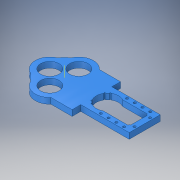
# Autodesk Inventor part: 000.401 - Опорная платформа
Saved by Autodesk Inventor 2019 (Build 230136000, 136)
## iProperties
Created: 2020-03-18
Part Number: 000.401 - Опорная платформа
Material: Пластик АБС
Document SubType Name: Modeling
Designer: Петров Иван
Density: 1.06 g/cm^3
Appearance: Голубой
Author: Петров Иван
Autodesk Inventor part; units mm, degrees
ref_plane "YZ Plane" through (0, 0, 0) normal (1, 0, 0) x (0, 1, 0)
ref_plane "XZ Plane" through (0, 0, 0) normal (0, 1, 0) x (-1, 0, 0)
ref_plane "XY Plane" through (0, 0, 0) normal (0, 0, 1) x (1, 0, 0)
sketch "Эскиз1" plane through (0, 0, 0) normal (0, 1, 0) x (-1, 0, 0)
  circle A0 centre (0, 0) radius 13.8
  circle A1 centre (-8, 0) radius 1.2
  circle A2 centre (0, -8) radius 1.2
  circle A3 centre (8, 0) radius 1.2
  circle A4 centre (0, 8) radius 1.2
  circle A5 centre (-7.7782, 7.7782) radius 1.2813
  circle A6 centre (-11, 0) radius 1.2813
  circle A7 centre (-7.7782, -7.7782) radius 1.2813
  circle A8 centre (0, -11) radius 1.2812
  circle A9 centre (7.7782, -7.7782) radius 1.2812
  circle A10 centre (11, 0) radius 1.2813
  circle A11 centre (7.7782, 7.7782) radius 1.2812
  circle A12 centre (0, 11) radius 1.2812
  circle A13 centre (0, 0) radius 5
  circle A14 centre (0, 0) radius 14
  circle A15 centre (0, 0) radius 1.55
  circle A16 centre (0, 0) radius 1.75
  circle A17 centre (0, 0) radius 25
  dimension "d0" = 50
  constraints: 18 centre point, 1 coincident
  measures "d0" diameter of A17
extrude "Выдавливание1" add sketch "Эскиз1" along normal blind 6 contours A0 | A1 | A2 | A3 | A4 | A5 | A6 | A7 | A8 | A9 | A10 | A11 | A12 | A13 | A14 | A15 | A16 | A17
sketch "Эскиз2" plane through (0, 6, 0) normal (0, 1, 0) x (1, 0, 0)
  line L0 (25, 0) -> (100, 0)
  circle A0 centre (100, 0) radius 25
  line L1 (50, 0) -> (50, -20)
  line L2 (50, 0) -> (50, 20)
  circle A1 centre (0, 0) radius 25 projected
  arc A2 (4.9455, 24.506) -> (95.0545, 24.506) centre (50, 247.5) ccw
  arc A3 (95.0545, -24.506) -> (4.9455, -24.506) centre (50, -247.5) ccw
  line L3 (100, 25) -> (0, 25)
  line L4 (0, -25) -> (100, -25)
  line L5 (50, 20) -> (50, 25)
  line L6 (50, -20) -> (50, -25)
  line L7 (50, 25) -> (50, -25)
  dimension "d3" = 100
  dimension "d4" = 50
  dimension "d5" = 20
  dimension "d6" = 20
  constraints: 16 end point, 15 point on circle, 3 centre point, 3 tangent, 2 midpoint, 2 vertical, 1 coincident, 1 collinear, 1 horizontal, 1 point on line
  measures "d3" distance of point (0, 0) L0.end
  measures "d4" diameter of A0
  measures "d5" distance of L1.start L1.end
  measures "d6" distance of L1.start L2.end
extrude "Выдавливание2" add sketch "Эскиз2" against normal blind 6 contours A1 A2 L2 L0 | L0 L1 A3 A1 | A1 L3 L5 A2 | A3 L6 L4 A1
sketch "Эскиз7" plane through (0, 6, 0) normal (0, 1, 0) x (1, 0, 0)
  line L0 (100, 0) -> (100, 15)
  line L1 (100, 0) -> (100, -15)
  circle A0 centre (100, 15) radius 3
  circle A1 centre (100, -15) radius 3
  line L2 (100, 0) -> (115, 0)
  circle A2 centre (115, 0) radius 3
  point P0 (0, 0)
  dimension "d23" = 15
  dimension "d24" = 15
  dimension "d25" = 6
  dimension "d26" = 6
  dimension "d27" = 15
  dimension "d28" = 6
  constraints: 6 end point, 3 centre point, 3 coincident, 2 vertical, 1 horizontal, 1 other
  measures "d23" distance of L0.start L0.end
  measures "d24" distance of L0.start L1.end
  measures "d25" diameter of A0
  measures "d26" diameter of A1
  measures "d27" distance of L0.start L2.end
  measures "d28" diameter of A2
extrude "Выдавливание7" [suppressed]
move faces "Перенос1" translate (33, 0, 0) faces at (50, 4, 8.3333)
sketch "Эскиз11" plane through (0, 6, 0) normal (0, 1, 0) x (1, 0, 0)
  line L0 (83, -25) -> (0, -25) projected
  line L1 (83, -25) -> (33, -25)
  line L2 (33, -25) -> (33, -16)
  line L3 (33, -16) -> (83, -16)
  line L4 (83, -16) -> (83, -25)
  point P0 (0, 0)
  dimension "d41" = 50
  dimension "d42" = 9
  constraints: 8 end point, 2 parallel, 1 horizontal, 1 perpendicular
  measures "d41" distance of L2.end L3.end
  measures "d42" distance of L1.end L2.end
extrude "Выдавливание11" cut sketch "Эскиз11" against normal blind 10
mirror "Зеркальное отражение2" about plane through (0, 0, 0) normal (0, 0, 1) of "Выдавливание11"
sketch "Эскиз12" plane through (0, 6, 0) normal (0, 1, 0) x (1, 0, 0)
  line L0 (37.45, -10) -> (75.5915, -10)
  line L1 (37.45, -10) -> (37.45, -11.4565)
  arc A0 (37.45, -11.4565) -> (38, -11.5) centre (38, -8) ccw
  line L2 (38, -11.5) -> (46.5, -11.5)
  line L3 (46.5, -11.5) -> (46.5, -13)
  line L4 (46.5, -13) -> (48, -13)
  line L5 (48, -13) -> (48, -15)
  line L6 (48, -15) -> (54.5, -15)
  line L7 (54.5, -15) -> (54.5, -13)
  line L8 (54.5, -13) -> (56, -13)
  line L9 (56, -13) -> (56, -15)
  line L10 (56, -15) -> (62.5, -15)
  line L11 (62.5, -15) -> (62.5, -13)
  line L12 (62.5, -13) -> (64, -13)
  line L13 (64, -13) -> (64, -15)
  line L14 (64, -15) -> (70.5, -15)
  line L15 (70.5, -15) -> (70.5, -13)
  line L16 (70.5, -13) -> (72, -13)
  line L17 (72, -13) -> (72, -15)
  line L18 (72, -15) -> (78.5, -15)
  line L19 (78.5, -15) -> (78.5, -13)
  line L20 (78.5, -13) -> (80, -13)
  line L21 (80, -13) -> (80, -11.25)
  line L22 (80, -11.25) -> (82, -11.25)
  line L23 (82, -11.25) -> (82, -4.75)
  line L24 (82, -4.75) -> (80, -4.75)
  line L25 (80, -4.75) -> (80, 4.75)
  line L26 (80, 4.75) -> (82, 4.75)
  line L27 (82, 4.75) -> (82, 11.25)
  line L28 (82, 11.25) -> (80, 11.25)
  line L29 (80, 11.25) -> (80, 13)
  line L30 (80, 13) -> (78.5, 13)
  line L31 (78.5, 13) -> (78.5, 15)
  line L32 (78.5, 15) -> (72, 15)
  line L33 (72, 15) -> (72, 13)
  line L34 (72, 13) -> (70.5, 13)
  line L35 (70.5, 13) -> (70.5, 15)
  line L36 (70.5, 15) -> (64, 15)
  line L37 (64, 15) -> (64, 13)
  line L38 (64, 13) -> (62.5, 13)
  line L39 (62.5, 13) -> (62.5, 15)
  line L40 (62.5, 15) -> (56, 15)
  line L41 (56, 15) -> (56, 13)
  line L42 (56, 13) -> (54.5, 13)
  line L43 (54.5, 13) -> (54.5, 15)
  line L44 (54.5, 15) -> (48, 15)
  line L45 (48, 15) -> (48, 13)
  line L46 (48, 13) -> (46.5, 13)
  line L47 (46.5, 13) -> (46.5, 11.5)
  line L48 (46.5, 11.5) -> (38, 11.5)
  arc A1 (38, 11.5) -> (37.4779, 11.4608) centre (38, 8) ccw
  line L49 (37.4779, 11.4608) -> (37.4779, 10)
  line L50 (75.5279, 10) -> (37.4779, 10)
  line L51 (75.5279, 10) -> (75.6016, 9.9543)
  arc A2 (76.9429, 8.5313) -> (75.6016, 9.9543) centre (77.5, 10.4) ccw
  line L52 (76.9429, 8.5313) -> (77, 8.4256)
  line L53 (77, -8.5152) -> (77, 8.4256)
  arc A3 (75.5915, -10) -> (77, -8.5152) centre (77.5, -10.4) ccw
  circle A4 centre (59.25, -13.5) radius 1.25
  circle A5 centre (75.25, -13.5) radius 1.25
  circle A6 centre (80.5, 8) radius 1.25
  circle A7 centre (75.25, 13.5) radius 1.25
  circle A8 centre (67.25, 13.5) radius 1.25
  circle A9 centre (59.25, 13.5) radius 1.25
  circle A10 centre (51.25, 13.5) radius 1.25
  circle A11 centre (80.5, -8) radius 1.25
  circle A12 centre (67.25, -13.5) radius 1.25
  circle A13 centre (51.25, -13.5) radius 1.25
  arc A14 (37.45, -9.25) -> (35.5, -7.3) centre (35.5, -9.25) ccw
  line L54 (37.45, -9.25) -> (37.45, -10)
  line L55 (37.45, -10) -> (53.45, -10)
  line L56 (53.45, -10) -> (53.25, -9.8)
  line L57 (53.25, -7.0711) -> (53.25, -9.8)
  arc A15 (53.25, -7.0711) -> (53.25, 7.0711) centre (44.5, 0) ccw
  line L58 (53.25, 9.8) -> (53.25, 7.0711)
  line L59 (53.25, 9.8) -> (53.45, 10)
  line L60 (53.45, 10) -> (37.45, 10)
  line L61 (37.45, 10) -> (37.45, 9.25)
  arc A16 (35.5, 7.3) -> (37.45, 9.25) centre (35.5, 9.25) ccw
  line L62 (35.5, 7.3) -> (34.5, 7.3)
  line L63 (34.5, 7.3) -> (34.5, -7.3)
  line L64 (34.5, -7.3) -> (35.5, -7.3)
  circle A17 centre (44.5, 0) radius 9.1
  line L65 (53.45, 10) -> (37.45, 10)
  line L66 (46.5, 13) -> (46.5, 11.5)
  line L67 (38, 13) -> (46.5, 13)
  line L68 (38, 11.5) -> (38, 13)
  line L69 (46.5, 11.5) -> (38, 11.5)
  arc A18 (38, 13) -> (37.4501, 12.9697) centre (38, 8) ccw
  spline S0 degree 3 poles (37.4501, 12.9697) (37.4501, 12.9689) (37.4503, 12.9605) (37.4503, 12.9597) (37.4503, 12.959) (37.4503, 12.9582) (37.4503, 12.9574) (37.4503, 12.9541) (37.4504, 12.9501) (37.4505, 12.9454) (37.4505, 12.9438) (37.4505, 12.9421) (37.4505, 12.9403) (37.4505, 12.9395) (37.4506, 12.9387) (37.4506, 12.9379) (37.4506, 12.9353) (37.4506, 12.9324) (37.4507, 12.9294) (37.4508, 12.9234) (37.4509, 12.9168) (37.451, 12.9095) (37.451, 12.9077) (37.451, 12.9059) (37.451, 12.9041) (37.4511, 12.8983) (37.4512, 12.8922) (37.4513, 12.8858) (37.4514, 12.8786) (37.4515, 12.8711) (37.4516, 12.8629) (37.4516, 12.8601) (37.4517, 12.8571) (37.4517, 12.8541) (37.4519, 12.8456) (37.452, 12.8366) (37.4521, 12.8272) (37.4523, 12.8162) (37.4524, 12.8046) (37.4526, 12.7924) (37.4528, 12.7801) (37.453, 12.7673) (37.4532, 12.7538) (37.4533, 12.7471) (37.4534, 12.7401) (37.4535, 12.7331) (37.4536, 12.7264) (37.4537, 12.7196) (37.4538, 12.7126) (37.454, 12.6978) (37.4542, 12.6823) (37.4545, 12.6664) (37.4547, 12.6528) (37.4549, 12.6387) (37.4551, 12.6244) (37.4553, 12.6118) (37.4555, 12.5991) (37.4557, 12.5862) (37.4558, 12.5798) (37.4559, 12.5734) (37.456, 12.5669) (37.4562, 12.5538) (37.4564, 12.5402) (37.4567, 12.5259) (37.457, 12.5031) (37.4574, 12.4796) (37.4578, 12.4556) (37.458, 12.4458) (37.4581, 12.4359) (37.4583, 12.4258) (37.4585, 12.4158) (37.4586, 12.4056) (37.4588, 12.3954) (37.4592, 12.3748) (37.4595, 12.354) (37.4599, 12.3329) (37.4601, 12.3203) (37.4603, 12.3076) (37.4605, 12.2948) (37.4607, 12.286) (37.4608, 12.2773) (37.461, 12.2685) (37.4614, 12.2466) (37.4618, 12.2245) (37.4622, 12.2021) (37.4624, 12.1909) (37.4626, 12.1796) (37.4628, 12.1683) (37.463, 12.1568) (37.4632, 12.1454) (37.4634, 12.1339) (37.4638, 12.1145) (37.4642, 12.0951) (37.4645, 12.0752) (37.4646, 12.0714) (37.4647, 12.0676) (37.4648, 12.0637) (37.4649, 12.0547) (37.4651, 12.0456) (37.4653, 12.0365) (37.4656, 12.0216) (37.4659, 12.0067) (37.4662, 11.9916) (37.4666, 11.9672) (37.4671, 11.9425) (37.4676, 11.9178) (37.4681, 11.8931) (37.4687, 11.8682) (37.4692, 11.8433) (37.4697, 11.8183) (37.4702, 11.7932) (37.4708, 11.7681) (37.4719, 11.7177) (37.473, 11.6669) (37.4742, 11.6157) (37.4754, 11.5645) (37.4766, 11.5128) (37.4779, 11.4608) knots 0.064201 0.064201 0.064201 0.064201 0.072529 0.072529 0.072529 0.080597 0.080597 0.080597 0.113423 0.113423 0.113423 0.125 0.125 0.125 0.12994 0.12994 0.12994 0.146482 0.146482 0.146482 0.17952 0.17952 0.17952 0.1875 0.1875 0.1875 0.212571 0.212571 0.212571 0.240274 0.240274 0.240274 0.25 0.25 0.25 0.277642 0.277642 0.277642 0.310147 0.310147 0.310147 0.342874 0.342874 0.342874 0.3593 0.3593 0.3593 0.375 0.375 0.375 0.408683 0.408683 0.408683 0.4375 0.4375 0.4375 0.462715 0.462715 0.462715 0.475013 0.475013 0.475013 0.5 0.5 0.5 0.540067 0.540067 0.540067 0.556372 0.556372 0.556372 0.572723 0.572723 0.572723 0.605497 0.605497 0.605497 0.625 0.625 0.625 0.638264 0.638264 0.638264 0.671081 0.671081 0.671081 0.6875 0.6875 0.6875 0.704131 0.704131 0.704131 0.732078 0.732078 0.732078 0.737463 0.737463 0.737463 0.75 0.75 0.75 0.770238 0.770238 0.770238 0.802948 0.802948 0.802948 0.835688 0.835688 0.835688 0.868461 0.868461 0.868461 0.93413 0.93413 0.93413 1 1 1 1
  arc A19 (38, 11.5) -> (37.4779, 11.4608) centre (38, 8) ccw
  line L70 (38, 11.5) -> (38, 13)
  arc A20 (37.4501, 12.9697) -> (33, 8) centre (38, 8) ccw
  line L71 (33, 7.3) -> (33, 8)
  line L72 (33, -7.3) -> (33, 7.3)
  line L73 (33, -8) -> (33, -7.3)
  arc A21 (33, -8) -> (37.4271, -12.9671) centre (38, -8) ccw
  line L74 (46.5, -13) -> (38, -13)
  arc A22 (37.4271, -12.9671) -> (38, -13) centre (38, -8) ccw
  line L75 (48, -16) -> (48, -15)
  line L76 (54.5, -16) -> (48, -16)
  line L77 (54.5, -15) -> (54.5, -16)
  line L78 (48, -15) -> (54.5, -15)
  line L79 (56, -16) -> (56, -15)
  line L80 (62.5, -16) -> (56, -16)
  line L81 (62.5, -15) -> (62.5, -16)
  line L82 (56, -15) -> (62.5, -15)
  line L83 (64, -16) -> (64, -15)
  line L84 (70.5, -16) -> (64, -16)
  line L85 (70.5, -15) -> (70.5, -16)
  line L86 (64, -15) -> (70.5, -15)
  line L87 (72, -16) -> (72, -15)
  line L88 (78.5, -16) -> (72, -16)
  line L89 (78.5, -15) -> (78.5, -16)
  line L90 (72, -15) -> (78.5, -15)
  line L91 (83, -11.25) -> (82, -11.25)
  line L92 (83, -4.75) -> (83, -11.25)
  line L93 (82, -4.75) -> (83, -4.75)
  line L94 (82, -11.25) -> (82, -4.75)
  line L95 (83, 4.75) -> (82, 4.75)
  line L96 (83, 11.25) -> (83, 4.75)
  line L97 (82, 11.25) -> (83, 11.25)
  line L98 (82, 4.75) -> (82, 11.25)
  line L99 (78.5, 16) -> (78.5, 15)
  line L100 (72, 16) -> (78.5, 16)
  line L101 (72, 15) -> (72, 16)
  line L102 (78.5, 15) -> (72, 15)
  line L103 (70.5, 16) -> (70.5, 15)
  line L104 (64, 16) -> (70.5, 16)
  line L105 (64, 15) -> (64, 16)
  line L106 (70.5, 15) -> (64, 15)
  line L107 (56, 16) -> (62.5, 16)
  line L108 (62.5, 16) -> (62.5, 15)
  line L109 (56, 16) -> (62.5, 16)
  line L110 (56, 15) -> (56, 16)
  line L111 (62.5, 15) -> (56, 15)
  line L112 (54.5, 16) -> (54.5, 15)
  line L113 (48, 16) -> (54.5, 16)
  line L114 (48, 15) -> (48, 16)
  line L115 (54.5, 15) -> (48, 15)
  spline S1 degree 3 poles (37.45, -11.4565) (37.4497, -11.4689) (37.4495, -11.4813) (37.4492, -11.4937) (37.4487, -11.5195) (37.4482, -11.5454) (37.4477, -11.5712) (37.4472, -11.5969) (37.4467, -11.6225) (37.4462, -11.6481) (37.4456, -11.6821) (37.4449, -11.716) (37.4443, -11.7496) (37.444, -11.7664) (37.4437, -11.7832) (37.4434, -11.7999) (37.443, -11.825) (37.4425, -11.85) (37.4421, -11.8749) (37.442, -11.8808) (37.4419, -11.8868) (37.4418, -11.8927) (37.4415, -11.9115) (37.4412, -11.9304) (37.4409, -11.9492) (37.4407, -11.9616) (37.4405, -11.9739) (37.4403, -11.986) (37.4401, -11.9983) (37.4399, -12.0104) (37.4397, -12.0224) (37.4396, -12.0258) (37.4396, -12.0292) (37.4395, -12.0327) (37.4392, -12.0531) (37.4389, -12.0734) (37.4386, -12.0936) (37.4379, -12.1324) (37.4374, -12.1706) (37.4368, -12.208) (37.4367, -12.2155) (37.4366, -12.2229) (37.4365, -12.2303) (37.4362, -12.2507) (37.4359, -12.2709) (37.4356, -12.2908) (37.4353, -12.3141) (37.435, -12.3369) (37.4346, -12.3594) (37.4345, -12.3699) (37.4343, -12.3802) (37.4342, -12.3905) (37.4341, -12.3973) (37.434, -12.4041) (37.4339, -12.4108) (37.4339, -12.4142) (37.4338, -12.4176) (37.4338, -12.421) (37.4336, -12.4356) (37.4334, -12.4501) (37.4332, -12.4643) (37.4331, -12.4696) (37.4331, -12.4747) (37.433, -12.4799) (37.4328, -12.4947) (37.4326, -12.509) (37.4324, -12.5227) (37.4324, -12.527) (37.4323, -12.5314) (37.4323, -12.5357) (37.432, -12.5537) (37.4318, -12.5714) (37.4316, -12.5885) (37.4314, -12.6056) (37.4312, -12.6223) (37.431, -12.6384) (37.4308, -12.6545) (37.4306, -12.6702) (37.4304, -12.6853) (37.4303, -12.6935) (37.4302, -12.7016) (37.4301, -12.7095) (37.43, -12.7161) (37.4299, -12.7227) (37.4298, -12.7291) (37.4298, -12.7362) (37.4297, -12.7431) (37.4296, -12.7499) (37.4295, -12.7567) (37.4294, -12.7633) (37.4293, -12.7697) (37.4293, -12.7755) (37.4292, -12.7811) (37.4291, -12.7866) (37.4291, -12.7934) (37.429, -12.8001) (37.4289, -12.8066) (37.4288, -12.8161) (37.4287, -12.8252) (37.4286, -12.8338) (37.4286, -12.8358) (37.4286, -12.8378) (37.4285, -12.8397) (37.4285, -12.8437) (37.4284, -12.8476) (37.4284, -12.8514) (37.4282, -12.8675) (37.428, -12.8819) (37.4279, -12.8948) (37.4278, -12.9027) (37.4277, -12.9101) (37.4276, -12.9167) (37.4276, -12.9234) (37.4275, -12.9295) (37.4274, -12.9349) (37.4274, -12.9403) (37.4273, -12.945) (37.4273, -12.949) (37.4272, -12.953) (37.4272, -12.9564) (37.4272, -12.9591) (37.4271, -12.9644) (37.4271, -12.9671) (37.4271, -12.9671) knots 0 0 0 0 0.015717 0.015717 0.015717 0.048574 0.048574 0.048574 0.081322 0.081322 0.081322 0.125 0.125 0.125 0.146869 0.146869 0.146869 0.179663 0.179663 0.179663 0.1875 0.1875 0.1875 0.212348 0.212348 0.212348 0.228682 0.228682 0.228682 0.245216 0.245216 0.245216 0.25 0.25 0.25 0.278672 0.278672 0.278672 0.333784 0.333784 0.333784 0.344755 0.344755 0.344755 0.375 0.375 0.375 0.410279 0.410279 0.410279 0.42665 0.42665 0.42665 0.4375 0.4375 0.4375 0.443003 0.443003 0.443003 0.466515 0.466515 0.466515 0.475131 0.475131 0.475131 0.5 0.5 0.5 0.507943 0.507943 0.507943 0.541148 0.541148 0.541148 0.574177 0.574177 0.574177 0.607119 0.607119 0.607119 0.625 0.625 0.625 0.640065 0.640065 0.640065 0.65654 0.65654 0.65654 0.672965 0.672965 0.672965 0.6875 0.6875 0.6875 0.705429 0.705429 0.705429 0.731487 0.731487 0.731487 0.737562 0.737562 0.737562 0.75 0.75 0.75 0.803346 0.803346 0.803346 0.83629 0.83629 0.83629 0.869201 0.869201 0.869201 0.902051 0.902051 0.902051 0.934818 0.934818 0.934818 1 1 1 1
  line L116 (37.25, -12.7684) -> (37.25, -11.4565)
  line L117 (37.25, -11.4565) -> (37.25, -10)
  line L118 (37.45, -10) -> (37.25, -10)
  line L119 (37.45, -11.4565) -> (37.25, -11.4565)
  line L120 (37.25, -12.7684) -> (37.25, -11.4565)
  line L121 (37.4271, -12.9671) -> (37.25, -12.7684)
  spline S2 degree 3 poles (37.45, -11.4565) (37.4497, -11.4689) (37.4495, -11.4813) (37.4492, -11.4937) (37.4487, -11.5195) (37.4482, -11.5454) (37.4477, -11.5712) (37.4472, -11.5969) (37.4467, -11.6225) (37.4462, -11.6481) (37.4456, -11.6821) (37.4449, -11.716) (37.4443, -11.7496) (37.444, -11.7664) (37.4437, -11.7832) (37.4434, -11.7999) (37.443, -11.825) (37.4425, -11.85) (37.4421, -11.8749) (37.442, -11.8808) (37.4419, -11.8868) (37.4418, -11.8927) (37.4415, -11.9115) (37.4412, -11.9304) (37.4409, -11.9492) (37.4407, -11.9616) (37.4405, -11.9739) (37.4403, -11.986) (37.4401, -11.9983) (37.4399, -12.0104) (37.4397, -12.0224) (37.4396, -12.0258) (37.4396, -12.0292) (37.4395, -12.0327) (37.4392, -12.0531) (37.4389, -12.0734) (37.4386, -12.0936) (37.438, -12.1324) (37.4374, -12.1706) (37.4368, -12.208) (37.4367, -12.2155) (37.4366, -12.2229) (37.4365, -12.2303) (37.4362, -12.2507) (37.4359, -12.2709) (37.4356, -12.2908) (37.4353, -12.3141) (37.435, -12.3369) (37.4346, -12.3594) (37.4345, -12.3699) (37.4344, -12.3802) (37.4342, -12.3905) (37.4341, -12.3973) (37.434, -12.4041) (37.4339, -12.4108) (37.4339, -12.4142) (37.4338, -12.4176) (37.4338, -12.421) (37.4336, -12.4356) (37.4334, -12.4501) (37.4332, -12.4643) (37.4331, -12.4696) (37.4331, -12.4747) (37.433, -12.4799) (37.4328, -12.4947) (37.4326, -12.509) (37.4324, -12.5227) (37.4324, -12.527) (37.4323, -12.5314) (37.4323, -12.5357) (37.432, -12.5537) (37.4318, -12.5714) (37.4316, -12.5885) (37.4314, -12.6056) (37.4312, -12.6223) (37.431, -12.6384) (37.4308, -12.6545) (37.4306, -12.6702) (37.4304, -12.6853) (37.4303, -12.6935) (37.4302, -12.7016) (37.4301, -12.7095) (37.43, -12.7161) (37.4299, -12.7227) (37.4298, -12.7291) (37.4298, -12.7362) (37.4297, -12.7431) (37.4296, -12.7499) (37.4295, -12.7567) (37.4294, -12.7633) (37.4294, -12.7697) (37.4293, -12.7755) (37.4292, -12.7811) (37.4292, -12.7866) (37.4291, -12.7934) (37.429, -12.8001) (37.4289, -12.8066) (37.4288, -12.8161) (37.4287, -12.8252) (37.4286, -12.8338) (37.4286, -12.8358) (37.4286, -12.8378) (37.4285, -12.8397) (37.4285, -12.8437) (37.4284, -12.8476) (37.4284, -12.8514) (37.4282, -12.8675) (37.428, -12.8819) (37.4279, -12.8948) (37.4278, -12.9027) (37.4277, -12.9101) (37.4277, -12.9167) (37.4276, -12.9234) (37.4275, -12.9295) (37.4275, -12.9349) (37.4274, -12.9403) (37.4273, -12.945) (37.4273, -12.949) (37.4272, -12.953) (37.4272, -12.9564) (37.4272, -12.9591) (37.4271, -12.9644) (37.4271, -12.9671) (37.4271, -12.9671) knots 0 0 0 0 0.015717 0.015717 0.015717 0.048574 0.048574 0.048574 0.081322 0.081322 0.081322 0.125 0.125 0.125 0.146869 0.146869 0.146869 0.179663 0.179663 0.179663 0.1875 0.1875 0.1875 0.212348 0.212348 0.212348 0.228682 0.228682 0.228682 0.245216 0.245216 0.245216 0.25 0.25 0.25 0.278672 0.278672 0.278672 0.333784 0.333784 0.333784 0.344755 0.344755 0.344755 0.375 0.375 0.375 0.410279 0.410279 0.410279 0.42665 0.42665 0.42665 0.4375 0.4375 0.4375 0.443003 0.443003 0.443003 0.466515 0.466515 0.466515 0.475131 0.475131 0.475131 0.5 0.5 0.5 0.507943 0.507943 0.507943 0.541148 0.541148 0.541148 0.574177 0.574177 0.574177 0.607119 0.607119 0.607119 0.625 0.625 0.625 0.640065 0.640065 0.640065 0.65654 0.65654 0.65654 0.672965 0.672965 0.672965 0.6875 0.6875 0.6875 0.705429 0.705429 0.705429 0.731487 0.731487 0.731487 0.737562 0.737562 0.737562 0.75 0.75 0.75 0.803346 0.803346 0.803346 0.83629 0.83629 0.83629 0.869201 0.869201 0.869201 0.902051 0.902051 0.902051 0.934818 0.934818 0.934818 1 1 1 1
  line L122 (37.25, -10) -> (37.45, -10)
  line L123 (37.25, -11.4565) -> (37.25, -10)
  line L124 (37.45, -11.4565) -> (37.25, -11.4565)
  line L125 (37.45, -10) -> (37.45, -11.4565)
  line L126 (37.25, 11.4608) -> (37.4779, 11.4608)
  spline S3 degree 3 poles (37.4501, 12.9697) (37.4501, 12.9689) (37.4503, 12.9605) (37.4503, 12.9597) (37.4503, 12.959) (37.4503, 12.9582) (37.4503, 12.9574) (37.4503, 12.9541) (37.4504, 12.9501) (37.4505, 12.9454) (37.4505, 12.9438) (37.4505, 12.9421) (37.4505, 12.9403) (37.4505, 12.9395) (37.4506, 12.9387) (37.4506, 12.9379) (37.4506, 12.9353) (37.4506, 12.9324) (37.4507, 12.9294) (37.4508, 12.9234) (37.4509, 12.9168) (37.451, 12.9095) (37.451, 12.9077) (37.451, 12.9059) (37.451, 12.9041) (37.4511, 12.8983) (37.4512, 12.8922) (37.4513, 12.8858) (37.4514, 12.8786) (37.4515, 12.8711) (37.4516, 12.8629) (37.4516, 12.8601) (37.4517, 12.8571) (37.4517, 12.8541) (37.4519, 12.8456) (37.452, 12.8366) (37.4521, 12.8272) (37.4523, 12.8162) (37.4524, 12.8046) (37.4526, 12.7924) (37.4528, 12.7801) (37.453, 12.7673) (37.4532, 12.7538) (37.4533, 12.7471) (37.4534, 12.7401) (37.4535, 12.7331) (37.4536, 12.7264) (37.4537, 12.7196) (37.4538, 12.7126) (37.454, 12.6978) (37.4542, 12.6823) (37.4545, 12.6664) (37.4547, 12.6528) (37.4549, 12.6387) (37.4551, 12.6244) (37.4553, 12.6118) (37.4555, 12.5991) (37.4557, 12.5862) (37.4558, 12.5798) (37.4559, 12.5734) (37.456, 12.5669) (37.4562, 12.5538) (37.4564, 12.5402) (37.4567, 12.5259) (37.457, 12.5031) (37.4574, 12.4796) (37.4578, 12.4556) (37.458, 12.4458) (37.4581, 12.4359) (37.4583, 12.4258) (37.4585, 12.4158) (37.4586, 12.4056) (37.4588, 12.3954) (37.4591, 12.3748) (37.4595, 12.354) (37.4599, 12.3329) (37.4601, 12.3203) (37.4603, 12.3076) (37.4605, 12.2948) (37.4607, 12.286) (37.4608, 12.2773) (37.461, 12.2685) (37.4614, 12.2466) (37.4618, 12.2245) (37.4622, 12.2021) (37.4624, 12.1909) (37.4626, 12.1796) (37.4628, 12.1683) (37.463, 12.1568) (37.4632, 12.1454) (37.4634, 12.1339) (37.4638, 12.1145) (37.4642, 12.0951) (37.4645, 12.0752) (37.4646, 12.0714) (37.4647, 12.0676) (37.4648, 12.0637) (37.4649, 12.0547) (37.4651, 12.0456) (37.4653, 12.0365) (37.4656, 12.0216) (37.4659, 12.0067) (37.4662, 11.9916) (37.4666, 11.9672) (37.4671, 11.9425) (37.4676, 11.9178) (37.4681, 11.8931) (37.4686, 11.8682) (37.4692, 11.8433) (37.4697, 11.8183) (37.4702, 11.7932) (37.4708, 11.7681) (37.4719, 11.7177) (37.473, 11.6669) (37.4742, 11.6157) (37.4754, 11.5645) (37.4766, 11.5128) (37.4779, 11.4608) knots 0.064201 0.064201 0.064201 0.064201 0.072529 0.072529 0.072529 0.080597 0.080597 0.080597 0.113423 0.113423 0.113423 0.125 0.125 0.125 0.12994 0.12994 0.12994 0.146482 0.146482 0.146482 0.17952 0.17952 0.17952 0.1875 0.1875 0.1875 0.212571 0.212571 0.212571 0.240274 0.240274 0.240274 0.25 0.25 0.25 0.277642 0.277642 0.277642 0.310147 0.310147 0.310147 0.342874 0.342874 0.342874 0.3593 0.3593 0.3593 0.375 0.375 0.375 0.408683 0.408683 0.408683 0.4375 0.4375 0.4375 0.462715 0.462715 0.462715 0.475013 0.475013 0.475013 0.5 0.5 0.5 0.540067 0.540067 0.540067 0.556372 0.556372 0.556372 0.572723 0.572723 0.572723 0.605497 0.605497 0.605497 0.625 0.625 0.625 0.638264 0.638264 0.638264 0.671081 0.671081 0.671081 0.6875 0.6875 0.6875 0.704131 0.704131 0.704131 0.732078 0.732078 0.732078 0.737463 0.737463 0.737463 0.75 0.75 0.75 0.770238 0.770238 0.770238 0.802948 0.802948 0.802948 0.835688 0.835688 0.835688 0.868461 0.868461 0.868461 0.93413 0.93413 0.93413 1 1 1 1
  line L127 (37.2706, 12.7443) -> (37.4501, 12.9697)
  line L128 (37.25, 12.7184) -> (37.2706, 12.7443)
  line L129 (37.25, 11.4608) -> (37.25, 12.7184)
  line L130 (37.4779, 10) -> (37.25, 10)
  line L131 (37.4779, 11.4608) -> (37.4779, 10)
  line L132 (37.25, 11.4608) -> (37.4779, 11.4608)
  line L133 (37.25, 10) -> (37.25, 11.4608)
  arc A23 (37.45, -11.4565) -> (38, -11.5) centre (38, -8) ccw
  spline S4 degree 3 poles (37.45, -11.4565) (37.4497, -11.4689) (37.4495, -11.4813) (37.4492, -11.4937) (37.4487, -11.5195) (37.4482, -11.5454) (37.4477, -11.5712) (37.4472, -11.5969) (37.4467, -11.6225) (37.4462, -11.6481) (37.4456, -11.6821) (37.4449, -11.716) (37.4443, -11.7496) (37.444, -11.7664) (37.4437, -11.7832) (37.4434, -11.7999) (37.443, -11.825) (37.4425, -11.85) (37.4421, -11.8749) (37.442, -11.8808) (37.4419, -11.8868) (37.4418, -11.8927) (37.4415, -11.9115) (37.4412, -11.9304) (37.4409, -11.9492) (37.4407, -11.9616) (37.4405, -11.9739) (37.4403, -11.986) (37.4401, -11.9983) (37.4399, -12.0104) (37.4397, -12.0224) (37.4396, -12.0258) (37.4396, -12.0292) (37.4395, -12.0327) (37.4392, -12.0531) (37.4389, -12.0734) (37.4386, -12.0936) (37.438, -12.1324) (37.4374, -12.1706) (37.4368, -12.208) (37.4367, -12.2155) (37.4366, -12.2229) (37.4365, -12.2303) (37.4362, -12.2507) (37.4359, -12.2709) (37.4356, -12.2908) (37.4353, -12.3141) (37.435, -12.3369) (37.4346, -12.3594) (37.4345, -12.3699) (37.4344, -12.3802) (37.4342, -12.3905) (37.4341, -12.3973) (37.434, -12.4041) (37.4339, -12.4108) (37.4339, -12.4142) (37.4338, -12.4176) (37.4338, -12.421) (37.4336, -12.4356) (37.4334, -12.4501) (37.4332, -12.4643) (37.4331, -12.4696) (37.4331, -12.4747) (37.433, -12.4799) (37.4328, -12.4947) (37.4326, -12.509) (37.4324, -12.5227) (37.4324, -12.527) (37.4323, -12.5314) (37.4323, -12.5357) (37.432, -12.5537) (37.4318, -12.5714) (37.4316, -12.5885) (37.4314, -12.6056) (37.4312, -12.6223) (37.431, -12.6384) (37.4308, -12.6545) (37.4306, -12.6702) (37.4304, -12.6853) (37.4303, -12.6935) (37.4302, -12.7016) (37.4301, -12.7095) (37.43, -12.7161) (37.4299, -12.7227) (37.4298, -12.7291) (37.4298, -12.7362) (37.4297, -12.7431) (37.4296, -12.7499) (37.4295, -12.7567) (37.4294, -12.7633) (37.4294, -12.7697) (37.4293, -12.7755) (37.4292, -12.7811) (37.4292, -12.7866) (37.4291, -12.7934) (37.429, -12.8001) (37.4289, -12.8066) (37.4288, -12.8161) (37.4287, -12.8252) (37.4286, -12.8338) (37.4286, -12.8358) (37.4286, -12.8378) (37.4285, -12.8397) (37.4285, -12.8437) (37.4284, -12.8476) (37.4284, -12.8514) (37.4282, -12.8675) (37.428, -12.8819) (37.4279, -12.8948) (37.4278, -12.9027) (37.4277, -12.9101) (37.4277, -12.9167) (37.4276, -12.9234) (37.4275, -12.9295) (37.4274, -12.9349) (37.4274, -12.9403) (37.4273, -12.945) (37.4273, -12.949) (37.4272, -12.953) (37.4272, -12.9564) (37.4272, -12.9591) (37.4271, -12.9644) (37.4271, -12.9671) (37.4271, -12.9671) knots 0 0 0 0 0.015717 0.015717 0.015717 0.048574 0.048574 0.048574 0.081322 0.081322 0.081322 0.125 0.125 0.125 0.146869 0.146869 0.146869 0.179663 0.179663 0.179663 0.1875 0.1875 0.1875 0.212348 0.212348 0.212348 0.228682 0.228682 0.228682 0.245216 0.245216 0.245216 0.25 0.25 0.25 0.278672 0.278672 0.278672 0.333784 0.333784 0.333784 0.344755 0.344755 0.344755 0.375 0.375 0.375 0.410279 0.410279 0.410279 0.42665 0.42665 0.42665 0.4375 0.4375 0.4375 0.443003 0.443003 0.443003 0.466515 0.466515 0.466515 0.475131 0.475131 0.475131 0.5 0.5 0.5 0.507943 0.507943 0.507943 0.541148 0.541148 0.541148 0.574177 0.574177 0.574177 0.607119 0.607119 0.607119 0.625 0.625 0.625 0.640065 0.640065 0.640065 0.65654 0.65654 0.65654 0.672965 0.672965 0.672965 0.6875 0.6875 0.6875 0.705429 0.705429 0.705429 0.731487 0.731487 0.731487 0.737562 0.737562 0.737562 0.75 0.75 0.75 0.803346 0.803346 0.803346 0.83629 0.83629 0.83629 0.869201 0.869201 0.869201 0.902051 0.902051 0.902051 0.934818 0.934818 0.934818 1 1 1 1
  arc A24 (37.4271, -12.9671) -> (38, -13) centre (38, -8) ccw
  line L134 (38, -13) -> (38, -11.5)
  line L135 (83, 4.75) -> (83, -4.75)
  circle A25 centre (77.5, 10.4) radius 1.95
  circle A26 centre (77.5, -10.4) radius 1.95
  line L136 (83, -16) -> (83, 16) projected
  circle A27 centre (44.5, 0) radius 11.5
  point P0 (44.5, 0)
  point P1 (33, 0)
  point P2 (33, 0)
  point P3 (83, 0)
  point P4 (83, 0)
  constraints: 272 end point, 28 point on circle, 26 centre point, 3 midpoint, 2 coincident, 1 point on line, 1 tangent, 16 other
extrude "Выдавливание13" cut sketch "Эскиз12" against normal blind 10 contours L56 L57 A27 L58 L59 L50 L51 A25 L52 L53 A26 L0 | L0 A27 L57 L56 | A27 L0 | L0 A27 A14 L63 A16 L50 L58 A15 L57 | L0 L54 A14 A27 | L57 A15 L58 A27 | A27 A14 | A14 L64 L63 A27 | A27 L50 L59 L58 | A27 L63 | L50 A27 | L63 L62 A16 A27 | A27 A16 L61 L60 L50 | A27 A16 | A4 | A5 | A6 | A7 | A8 | A9 | A10 | A11 | A12 | A13 | A17
sketch "Эскиз13" plane through (0, 6, 0) normal (0, 1, 0) x (1, 0, 0)
  circle A0 centre (-14.1421, -14.1421) radius 2.1
  circle A1 centre (10, 0) radius 2.1
  circle A2 centre (-14.1421, 14.1421) radius 2.1
  circle A3 centre (-15.0247, 0.005) radius 9.5
  circle A4 centre (-0.0247, 15.005) radius 9.5
  circle A5 centre (-0.0247, -14.995) radius 9.5
  line L0 (13.7779, -24.9956) -> (13.7779, 25.0044)
  line L1 (13.7779, 25.0044) -> (-0.0275, 25.0044)
  arc A6 (-0.0275, 25.0044) -> (-0.0275, -24.9956) centre (-0.0275, 0.0044) ccw
  line L2 (-0.0275, -24.9956) -> (13.7779, -24.9956)
  point P0 (0, 0)
  point P1 (0, 0)
  constraints: 7 centre point, 6 end point, 2 point on circle
extrude "Выдавливание14" cut sketch "Эскиз13" against normal blind 10 contours A3 | A4 | A5
sketch "Эскиз14" plane through (0, 6, 0) normal (0, 1, 0) x (1, 0, 0)
  circle A0 centre (-0.0247, 15.005) radius 9.5 projected
  arc A1 (-5.585, 1.0736) -> (-13.956, 9.4447) centre (-0.0247, 15.005) ccw
  circle A2 centre (-0.0247, -14.995) radius 9.5 projected
  arc A3 (-13.9504, -9.4341) -> (-5.5856, -1.0692) centre (-0.0247, -14.995) ccw
  circle A4 centre (-15.0247, 0.005) radius 9.5 projected
  arc A5 (-9.4675, 13.9642) -> (-9.4675, -13.9542) centre (-15.0247, 0.005) ccw
  arc A6 (-1.0655, -5.5522) -> (-1.0655, 5.5622) centre (-15.0247, 0.005) ccw
  point P0 (0, 0)
  dimension "d52" = 30
  constraints: 18 point on circle, 4 centre point, 3 coincident
  measures "d52" diameter of A1
extrude "Выдавливание15" add sketch "Эскиз14" against normal blind 6 contours A0 A5 A1 A6 | A0 A6 A1 A4 A5 | A1 A4 A3 A5 | A6 A3 A4 A1 | A5 A2 A6 A3 | A3 A4 A6 A2 A5
equation "\"d6\" = d5"
equation "\"d24\" = d23"
equation "\"d26\" = d25"
equation "\"d27\" = d23"
equation "\"d28\" = d25"
